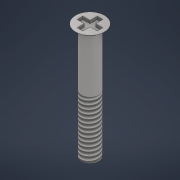
# Autodesk Inventor part: Parafuso
Saved by Autodesk Inventor 2021 (Build 250183000, 183)
## iProperties
Created: 2021-01-20
Part Number: Parafuso
Material: Genérico
Document SubType Name: Modeling
Designer: João
Density: 1 g/cm^3
Appearance: Padrão
Author: João
Autodesk Inventor part; units mm, degrees
ref_plane "YZ Plane" through (0, 0, 0) normal (1, 0, 0) x (0, 1, 0)
ref_plane "XZ Plane" through (0, 0, 0) normal (0, 1, 0) x (-1, 0, 0)
sketch "Esboço1" plane through (0, 0, 0) normal (0, 1, 0) x (-1, 0, 0)
  circle A0 centre (0, 0) radius 0.75
  dimension "d1" = 1.5
  constraints: 1 centre point
  measures "d1" diameter of A0
extrude "Extrusão1" add sketch "Esboço1" along normal blind 9.6
ref_plane "Plano de trabalho1" through (0, 10, 0) normal (0, 1, 0) x (1, 0, 0)
sketch "Esboço2" plane through (0, 10, 0) normal (0, 1, 0) x (1, 0, 0)
  circle A0 centre (0, 0) radius 1.25
  dimension "d5" = 2.5
  constraints: 1 centre point, 1 coincident
  measures "d5" diameter of A0
loft "Transição1" add profiles "Esboço2" section 1 edges at (0.75, 9.6, 0)
sketch "Esboço3" plane through (0, 10, 0) normal (0, 1, 0) x (1, 0, 0)
  line L0 (0.25, -0.875) -> (-0.25, -0.875)
  line L1 (-0.25, -0.875) -> (-0.25, 0.875)
  line L2 (-0.25, 0.875) -> (0.25, 0.875)
  line L3 (0.25, 0.875) -> (0.25, -0.875)
  line L4 (0.25, -0.875) -> (-0.25, 0.875) construction
  line L5 (-0.25, -0.875) -> (0.25, 0.875) construction
  line L6 (-0.875, -0.25) -> (0.875, -0.25)
  line L7 (0.875, -0.25) -> (0.875, 0.25)
  line L8 (0.875, 0.25) -> (-0.875, 0.25)
  line L9 (-0.875, 0.25) -> (-0.875, -0.25)
  line L10 (-0.875, -0.25) -> (0.875, 0.25) construction
  line L11 (0.875, -0.25) -> (-0.875, 0.25) construction
  point P0 (0, 0)
  point P1 (-0.25, 0.25)
  point P2 (-0.25, -0.25)
  point P3 (0.25, -0.25)
  point P4 (0.25, 0.25)
  dimension "d10" = 0.5
  dimension "d11" = 1.75
  dimension "d14" = 1.75
  dimension "d15" = 0.5
  constraints: 24 end point, 4 midpoint, 4 parallel, 2 horizontal, 2 perpendicular
  measures "d10" distance of L1.end L2.end
  measures "d11" distance of L0.end L1.end
  measures "d14" distance of L8.end L7.end
  measures "d15" distance of L7.end L6.end
extrude "Extrusão2" cut sketch "Esboço3" against normal blind 0.25
thread "Rosca1" size "M1.6x0.35" class "6g" standard "ANSI Metric M Profile" length 5
